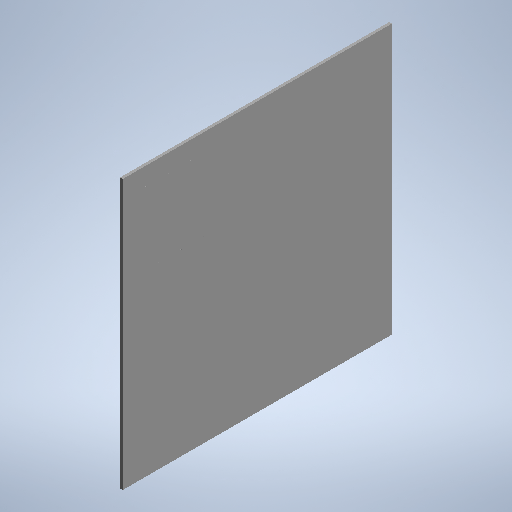
# Autodesk Inventor part: RT_FRM_MC_009_ElectricalBackPlate_Inside
Saved by Autodesk Inventor 2025.4 (Build 294407000, 407)
## iProperties
Created: 2026-05-16
Part Number: RT_FRM_MC_009_ElectricalBackPlate_Inside
Material: Générique
Document SubType Name: Modeling
Designer: louis
Density: 1 g/cm^3
Appearance: Par défaut
Author: louis
Autodesk Inventor part; units mm, degrees
ref_plane "YZ Plane" through (0, 0, 0) normal (1, 0, 0) x (0, 1, 0)
ref_plane "XZ Plane" through (0, 0, 0) normal (0, 1, 0) x (-1, 0, 0)
ref_plane "XY Plane" through (0, 0, 0) normal (0, 0, 1) x (1, 0, 0)
sketch "Sketch2" plane through (0, 0, 0) normal (1, 0, 0) x (0, 1, 0)
  line L0 (-300, -300) -> (300, -300)
  line L1 (300, -300) -> (300, 300)
  line L2 (300, 300) -> (-300, 300)
  line L3 (-300, 300) -> (-300, -300)
  line L4 (-300, -300) -> (300, 300) construction
  line L5 (300, -300) -> (-300, 300) construction
  point P0 (0, 0)
  dimension "d0" = 600
  dimension "d1" = 600
  constraints: 12 end point, 2 midpoint, 2 parallel, 1 horizontal, 1 perpendicular
  measures "d0" distance of L2.end L1.end
  measures "d1" distance of L1.end L0.end
extrude "Extrusion1" add sketch "Sketch2" along normal blind 6
sketch "Sketch3" plane through (6, 0, 0) normal (1, 0, 0) x (0, 0, -1)
  line L0 (0, 0) -> (-260, 0) construction
  line L1 (-260, 0) -> (-260, -248) construction
  line L2 (-99, 0) -> (-99, -248) construction
  line L3 (-99, -248) -> (-260, -248) construction
  line L4 (-260, -220) -> (-99, -220) construction
  line L5 (-264.5, -254) -> (-94.5, -254) construction
  line L6 (-94.5, -254) -> (-94.5, -214) construction
  line L7 (-94.5, -214) -> (-264.5, -214) construction
  line L8 (-264.5, -214) -> (-264.5, -254) construction
  line L9 (-179.5, -254) -> (-179.5, -248) construction
  line L10 (-179.5, -220) -> (-179.5, -214) construction
  dimension "d13" = 161
  dimension "d14" = 28
  dimension "d15" = 220
  dimension "d16" = 260
  dimension "d17" = 40
  dimension "d18" = 170
  constraints: 22 end point, 5 perpendicular, 4 midpoint, 3 point on line, 2 coincident, 2 horizontal, 2 parallel, 1 collinear, 1 vertical
  measures "d13" distance of L2.end L1.end
  measures "d14" distance between parallel lines of L4 L3
  measures "d15" distance from line of L0 L4.end
  measures "d16" distance of L0.start L0.end
  measures "d17" distance of L5.end L6.end
  measures "d18" distance of L5.start L5.end
hole "Hole1" at (6, -248, 260) at (6, -220, 99) direction (-1, 0, 0) diameter 3 end through all
pattern_linear "Rectangular Pattern1" count 3 spacing 50 along (0, 1, 0) of "Hole1"
body "Solid1"
